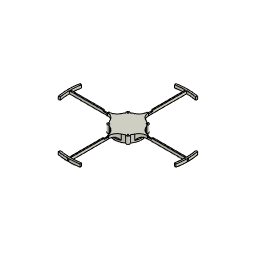
SoporteImán Nube Flotante v1 (Autodesk Fusion 360 design; units mm, degrees)
Autodesk Fusion 360 part; units mm, degrees
note: some values were not read from the file. Set by a fixed rule: which face or edge a step refers to.
sketch "Boceto1" plane through (0, 0, 0) normal (0, 0, 1) x (1, 0, 0)
  circle A0 centre (0, 0) radius 22.075
  circle A1 centre (0, 0) radius 24.075
  dimension "d1" = 44.15
  dimension "d2" = 2
  constraint coincident A0.centre A1.centre
  measures "d1" diameter of A0
extrude "Extruir1" add sketch "Boceto1" along normal blind 8 makes body 1
sketch "Boceto2" plane through (0, 0, 8) normal (0, 0, 1) x (-1, 0, 0)
  circle A0 centre (0, 0) radius 22.075
  circle A1 centre (0, 0) radius 24.075
  line L0 (0, 0) -> (-22.075, 0)
  line L1 (-22.075, 0) -> (-72.075, 0)
  line L2 (0, 0) -> (22.075, 0)
  line L3 (22.075, 0) -> (72.075, 0)
  line L4 (0, -22.075) -> (0, -72.075)
  line L5 (0, 22.075) -> (0, 72.075)
  line L6 (1, 22.075) -> (1, 72.075)
  line L7 (-1, 22.075) -> (-1, 72.075)
  line L8 (22.075, -1) -> (72.075, -1)
  line L9 (22.075, 1) -> (72.075, 1)
  line L10 (0, 1) -> (22.075, 1)
  line L11 (0, 1) -> (-22.075, 1)
  line L12 (-22.075, 1) -> (-72.075, 1)
  line L13 (-22.075, -1) -> (-72.075, -1)
  line L14 (1, -22.075) -> (1, -72.075)
  line L15 (-1, -22.075) -> (-1, -72.075)
  line L16 (72.075, 1) -> (72.075, -1)
  line L17 (1, 72.075) -> (-1, 72.075)
  line L18 (-72.075, 1) -> (-72.075, -1)
  line L19 (1, -72.075) -> (-1, -72.075)
  dimension "d7" = 50
  dimension "d8" = 50
  dimension "d9" = 50
  dimension "d10" = 50
  dimension "d11" = 1
  dimension "d12" = -1
  dimension "d13" = 1
  dimension "d14" = -1
  dimension "d15" = -1
  dimension "d16" = -1
  dimension "d17" = 1
  constraint coincident A0.centre A1.centre
  constraint coincident A0 L0.end
  constraint horizontal L0
  constraint parallel L0 L1
  constraint coincident A0 L2.end
  constraint parallel L0 L2
  constraint parallel L2 L3
  constraint coincident A0 L4.start
  constraint perpendicular L0 L4
  constraint coincident A0 L5.start
  constraint perpendicular L0 L5
  constraint perpendicular L8 L16
  constraint perpendicular L5 L17
  constraint perpendicular L13 L18
  constraint perpendicular L15 L19
  measures "d7" distance of L0.end L1.end
  measures "d8" distance of L2.end L3.end
  measures "d9" distance of L4.start L4.end
  measures "d10" distance of L5.start L5.end
extrude "Extruir2" add sketch "Boceto2" along normal blind 1 contours A0 L0 L2 | A0 A1 L1 L11 L12 | A0 L0 L2 L10 L11 | A0 A1 L1 L4 | A0 A1 L3 L4 | A0 A1 L5 L11 L12 | A0 L10 L11 | A0 A1 L3 L9 L10 | A0 A1 L5 L9 L10 bodies 1
extrude "Extruir4" add sketch "Boceto2" along normal blind 1 contours A1 L5 L6 L17 | A1 L5 L7 L17 bodies 1
extrude "Extruir5" add sketch "Boceto2" along normal blind 1 contours A1 L1 L12 L18 | A1 L1 L13 L18 | A1 L4 L15 L19 | A1 L4 L14 L19 | A1 L3 L8 L16 | A1 L3 L9 L16 bodies 1
sketch "Boceto3" plane through (0, 0, 9) normal (0, 0, 1) x (-1, 0, 0)
  arc A0 (-1, 24.0542) -> (-24.0542, 1) centre (0, 0) ccw
  line L0 (-24.0542, 1) -> (-72.075, 1)
  line L1 (-72.075, 1) -> (-72.075, -1)
  line L2 (-72.075, -1) -> (-24.0542, -1)
  arc A1 (-24.0542, -1) -> (-1, -24.0542) centre (0, 0) ccw
  line L3 (-1, -24.0542) -> (-1, -72.075)
  line L4 (-1, -72.075) -> (1, -72.075)
  line L5 (1, -72.075) -> (1, -24.0542)
  arc A2 (1, -24.0542) -> (24.0542, -1) centre (0, 0) ccw
  line L6 (24.0542, -1) -> (72.075, -1)
  line L7 (72.075, -1) -> (72.075, 1)
  line L8 (72.075, 1) -> (24.0542, 1)
  arc A3 (24.0542, 1) -> (1, 24.0542) centre (0, 0) ccw
  line L9 (1, 24.0542) -> (1, 72.075)
  line L10 (1, 72.075) -> (-1, 72.075)
  line L11 (-1, 72.075) -> (-1, 24.0542)
  circle A4 centre (0, 0) radius 24
  line L12 (0, 0) -> (16.2635, 16.2635)
  line L13 (0, 0) -> (23, 0) construction
  line L14 (16.2635, 16.2635) -> (-16.9706, -16.9706)
  line L15 (0, 0) -> (-16.9706, 16.9706)
  line L16 (-16.9706, 16.9706) -> (16.9706, -16.9706)
  circle A5 centre (-16.9706, 16.9706) radius 2
  circle A6 centre (16.2635, 16.2635) radius 2
  circle A7 centre (-16.9706, -16.9706) radius 2
  circle A8 centre (16.9706, -16.9706) radius 2
  dimension "d24" = 48
  dimension "d25" = 45
  dimension "d26" = 4
  dimension "d27" = 4
  dimension "d28" = 4
  dimension "d29" = 4
  constraint coincident A0.centre A1.centre
  constraint horizontal L13
  constraint coincident A4 L14.end
  constraint parallel L12 L14
  constraint coincident A4 L15.end
  constraint perpendicular L14 L15
  constraint coincident A4 L16.end
  constraint parallel L15 L16
  constraint coincident L15.end L16.start
  constraint coincident L12.end L14.start
  constraint coincident L14.end A7.centre
  constraint coincident L16.end A8.centre
  measures "d24" diameter of A4
  measures "d25" angle of L12 L13
  measures "d26" diameter of A5
  measures "d27" diameter of A6
  measures "d28" diameter of A7
  measures "d29" diameter of A8
extrude "Extruir6" add sketch "Boceto3" against normal blind 9 contours A0 A5 | A3 A6 | A1 A7 | A2 A8 bodies 1
sketch "Boceto4" plane through (0, 0, 9) normal (0, 0, 1) x (-1, 0, 0)
  arc A0 (-1, 24.0542) -> (-15.5506, 18.379) centre (0, 0) ccw
  arc A1 (-15.5506, 18.379) -> (-18.379, 15.5506) centre (-16.9706, 16.9706) ccw
  arc A2 (-18.379, 15.5506) -> (-24.0542, 1) centre (0, 0) ccw
  line L0 (-24.0542, 1) -> (-72.075, 1)
  line L1 (-72.075, 1) -> (-72.075, -1)
  line L2 (-72.075, -1) -> (-24.0542, -1)
  arc A3 (-24.0542, -1) -> (-18.379, -15.5506) centre (0, 0) ccw
  arc A4 (-18.379, -15.5506) -> (-15.5506, -18.379) centre (-16.9706, -16.9706) ccw
  arc A5 (-15.5506, -18.379) -> (-1, -24.0542) centre (0, 0) ccw
  line L3 (-1, -24.0542) -> (-1, -72.075)
  line L4 (-1, -72.075) -> (1, -72.075)
  line L5 (1, -72.075) -> (1, -24.0542)
  arc A6 (1, -24.0542) -> (15.5506, -18.379) centre (0, 0) ccw
  arc A7 (15.5506, -18.379) -> (18.379, -15.5506) centre (16.9706, -16.9706) ccw
  arc A8 (18.379, -15.5506) -> (24.0542, -1) centre (0, 0) ccw
  line L6 (24.0542, -1) -> (72.075, -1)
  line L7 (72.075, -1) -> (72.075, 1)
  line L8 (72.075, 1) -> (24.0542, 1)
  arc A9 (24.0542, 1) -> (18.1992, 15.7605) centre (0, 0) ccw
  arc A10 (18.1992, 15.7605) -> (15.7605, 18.1992) centre (16.2635, 16.2635) ccw
  arc A11 (15.7605, 18.1992) -> (1, 24.0542) centre (0, 0) ccw
  line L9 (1, 24.0542) -> (1, 72.075)
  line L10 (1, 72.075) -> (-1, 72.075)
  line L11 (-1, 72.075) -> (-1, 24.0542)
  circle A12 centre (-16.9706, -16.9706) radius 1.05
  circle A13 centre (16.9706, -16.9706) radius 1.05
  circle A14 centre (16.2635, 16.2635) radius 1.05
  circle A15 centre (-16.9706, 16.9706) radius 1.05
  dimension "d32" = 2.1
  dimension "d33" = 2.1
  dimension "d34" = 2.1
  dimension "d35" = 2.1
  constraint concentric A4 A12
  constraint concentric A7 A13
  constraint concentric A10 A14
  constraint concentric A1 A15
  measures "d32" diameter of A12
  measures "d33" diameter of A13
  measures "d34" diameter of A14
  measures "d35" diameter of A15
extrude "Extruir7" cut sketch "Boceto4" against normal blind 8 contours A12 | A13 | A14 | A15 bodies 1
extrude "Extruir8" add 1 faces at (-16.0835, -16.0654, 1) along direction (0, 0, 1) blind 120 separate body on bodies 1 makes body 2
extrude "Extruir9" add 1 faces at (-17.2533, 17.0815, 1) along direction (0, 0, 1) blind 120 separate body on bodies 1 makes body 3
extrude "Extruir10" add 1 faces at (16.6878, 17.0815, 1) along direction (0, 0, 1) blind 120 separate body on bodies 1 makes body 4
extrude "Extruir11" add 1 faces at (16.6878, -16.8596, 1) along direction (0, 0, 1) blind 120 separate body on bodies 1 makes body 5
sketch "Boceto5" plane through (0, 0, 9) normal (0, 0, 1) x (-1, 0, 0)
  circle A0 centre (-16.9706, -16.9706) radius 1.05
  circle A1 centre (16.9706, -16.9706) radius 1.05
  circle A2 centre (-16.9706, 16.9706) radius 1.05
  circle A3 centre (16.2635, 16.2635) radius 1.05
  arc A4 (-1, 24.0542) -> (-15.5506, 18.379) centre (0, 0) ccw
  arc A5 (-15.5506, 18.379) -> (-18.379, 15.5506) centre (-16.9706, 16.9706) ccw
  arc A6 (-18.379, 15.5506) -> (-24.0542, 1) centre (0, 0) ccw
  line L0 (-24.0542, 1) -> (-72.075, 1)
  line L1 (-72.075, 1) -> (-72.075, -1)
  line L2 (-72.075, -1) -> (-24.0542, -1)
  arc A7 (-24.0542, -1) -> (-18.379, -15.5506) centre (0, 0) ccw
  arc A8 (-18.379, -15.5506) -> (-15.5506, -18.379) centre (-16.9706, -16.9706) ccw
  arc A9 (-15.5506, -18.379) -> (-1, -24.0542) centre (0, 0) ccw
  line L3 (-1, -24.0542) -> (-1, -72.075)
  line L4 (-1, -72.075) -> (1, -72.075)
  line L5 (1, -72.075) -> (1, -24.0542)
  arc A10 (1, -24.0542) -> (15.5506, -18.379) centre (0, 0) ccw
  arc A11 (15.5506, -18.379) -> (18.379, -15.5506) centre (16.9706, -16.9706) ccw
  arc A12 (18.379, -15.5506) -> (24.0542, -1) centre (0, 0) ccw
  line L6 (24.0542, -1) -> (72.075, -1)
  line L7 (72.075, -1) -> (72.075, 1)
  line L8 (72.075, 1) -> (24.0542, 1)
  arc A13 (24.0542, 1) -> (18.1992, 15.7605) centre (0, 0) ccw
  arc A14 (18.1992, 15.7605) -> (15.7605, 18.1992) centre (16.2635, 16.2635) ccw
  arc A15 (15.7605, 18.1992) -> (1, 24.0542) centre (0, 0) ccw
  line L9 (1, 24.0542) -> (1, 72.075)
  line L10 (1, 72.075) -> (-1, 72.075)
  line L11 (-1, 72.075) -> (-1, 24.0542)
  circle A16 centre (0, 0) radius 24.075
  constraint coincident A4.centre A6.centre
  constraint coincident A11.end A16
extrude "Extruir12" add sketch "Boceto5" along normal blind 1 separate body contours A0 A1 A2 A4 A6 A7 A9 A10 A12 A13 A15 A16 | A0 A8 A16 | A2 A5 A16 | A1 A11 A16 | A14 A16 makes body 6
move_body "Desplazar1" bodies 6 to x (1, 0, 0) y (0, 1, 0) z (0, 0, 1) at (0, 0, 100)
sketch "Boceto6" plane through (0, 0, 110) normal (0, 0, 1) x (-1, 0, 0)
  circle A0 centre (-16.9706, 16.9706) radius 1.05
  circle A1 centre (16.2635, 16.2635) radius 1.05
  circle A2 centre (-16.9706, -16.9706) radius 1.05
  circle A3 centre (16.9706, -16.9706) radius 1.05
  arc A4 (18.379, -15.5506) -> (18.1992, 15.7605) centre (0, 0) ccw
  arc A5 (18.1992, 15.7605) -> (15.7605, 18.1992) centre (16.2635, 16.2635) ccw
  arc A6 (15.7605, 18.1992) -> (-15.5506, 18.379) centre (0, 0) ccw
  arc A7 (-15.5506, 18.379) -> (-18.379, 15.5506) centre (-16.9706, 16.9706) ccw
  arc A8 (-18.379, 15.5506) -> (-18.379, -15.5506) centre (0, 0) ccw
  arc A9 (-18.379, -15.5506) -> (-15.5506, -18.379) centre (-16.9706, -16.9706) ccw
  arc A10 (-15.5506, -18.379) -> (15.5506, -18.379) centre (0, 0) ccw
  arc A11 (15.5506, -18.379) -> (18.379, -15.5506) centre (16.9706, -16.9706) ccw
  circle A12 centre (0, 0) radius 20
  dimension "d48" = 40
  constraint coincident A4.centre A6.centre
  measures "d48" diameter of A12
extrude "Extruir13" cut sketch "Boceto6" against normal blind 1 contours A12 bodies 6
fillet "Empalme1" radius 15 1 edges at (-24.0542, 1, 8.5) on bodies 1
fillet "Empalme2" radius 15 1 edges at (-24.0542, -1, 8.5) on bodies 1
fillet "Empalme3" radius 15 2 edges at (-1, 24.0542, 8.5) (1, 24.0542, 8.5) on bodies 1
fillet "Empalme4" radius 15 4 edges at (24.0542, 1, 8.5) (24.0542, -1, 8.5) (1, -24.0542, 8.5) (-1, -24.0542, 8.5) on bodies 1
extrude "Extruir14" add 1 faces at (72.075, -0.3333, 8.3333) along direction (1, 0, 0) blind 20 on bodies 1 bodies 1
extrude "Extruir15" add 1 faces at (-0.3333, -72.075, 8.3333) along direction (0, -1, 0) blind 20 on bodies 1 bodies 1
extrude "Extruir16" add 1 faces at (-72.075, -0.3333, 8.3333) along direction (-1, 0, 0) blind 20 on bodies 1 bodies 1
extrude "Extruir17" add 1 faces at (-0.3333, 72.075, 8.3333) along direction (0, 1, 0) blind 20 on bodies 1 bodies 1
fillet "Empalme5" radius 5 1 edges at (-24.075, 0, 8) on bodies 1
fillet "Empalme6" radius 5 1 edges at (0, -24.075, 8) on bodies 1
fillet "Empalme7" radius 5 1 edges at (24.075, 0, 8) on bodies 1
fillet "Empalme8" radius 5 1 edges at (0, 24.075, 8) on bodies 1
extrude "Extruir18" add 1 faces at (-5.096, 5.6045, 9) along direction (0, 0, 1) blind 2 on bodies 1 bodies 1
sketch "Boceto7" plane through (0, 0, 11) normal (0, 0, 1) x (-1, 0, 0)
  circle A0 centre (-16.9706, -16.9706) radius 1.05
  circle A1 centre (16.9706, -16.9706) radius 1.05
  circle A2 centre (-16.9706, 16.9706) radius 1.05
  circle A3 centre (16.2635, 16.2635) radius 1.05
  arc A4 (-9.858, 21.9642) -> (-15.5506, 18.379) centre (0, 0) ccw
  arc A5 (-15.5506, 18.379) -> (-18.379, 15.5506) centre (-16.9706, 16.9706) ccw
  arc A6 (-18.379, 15.5506) -> (-21.9642, 9.858) centre (0, 0) ccw
  arc A7 (-35.6491, 1) -> (-21.9642, 9.858) centre (-35.6491, 16) ccw
  line L0 (-35.6491, 1) -> (-92.075, 1)
  line L1 (-92.075, 1) -> (-92.075, -1)
  line L2 (-92.075, -1) -> (-35.6491, -1)
  arc A8 (-21.9642, -9.858) -> (-35.6491, -1) centre (-35.6491, -16) ccw
  arc A9 (-21.9642, -9.858) -> (-18.379, -15.5506) centre (0, 0) ccw
  arc A10 (-18.379, -15.5506) -> (-15.5506, -18.379) centre (-16.9706, -16.9706) ccw
  arc A11 (-15.5506, -18.379) -> (-9.858, -21.9642) centre (0, 0) ccw
  arc A12 (-1, -35.6491) -> (-9.858, -21.9642) centre (-16, -35.6491) ccw
  line L3 (-1, -35.6491) -> (-1, -92.075)
  line L4 (-1, -92.075) -> (1, -92.075)
  line L5 (1, -92.075) -> (1, -35.6491)
  arc A13 (9.858, -21.9642) -> (1, -35.6491) centre (16, -35.6491) ccw
  arc A14 (9.858, -21.9642) -> (15.5506, -18.379) centre (0, 0) ccw
  arc A15 (15.5506, -18.379) -> (18.379, -15.5506) centre (16.9706, -16.9706) ccw
  arc A16 (18.379, -15.5506) -> (21.9642, -9.858) centre (0, 0) ccw
  arc A17 (35.6491, -1) -> (21.9642, -9.858) centre (35.6491, -16) ccw
  line L6 (35.6491, -1) -> (92.075, -1)
  line L7 (92.075, -1) -> (92.075, 1)
  line L8 (92.075, 1) -> (35.6491, 1)
  arc A18 (21.9642, 9.858) -> (35.6491, 1) centre (35.6491, 16) ccw
  arc A19 (21.9642, 9.858) -> (18.1992, 15.7605) centre (0, 0) ccw
  arc A20 (18.1992, 15.7605) -> (15.7605, 18.1992) centre (16.2635, 16.2635) ccw
  arc A21 (15.7605, 18.1992) -> (9.858, 21.9642) centre (0, 0) ccw
  arc A22 (1, 35.6491) -> (9.858, 21.9642) centre (16, 35.6491) ccw
  line L9 (1, 35.6491) -> (1, 92.075)
  line L10 (1, 92.075) -> (-1, 92.075)
  line L11 (-1, 92.075) -> (-1, 35.6491)
  arc A23 (-9.858, 21.9642) -> (-1, 35.6491) centre (-16, 35.6491) ccw
  circle A24 centre (16.9706, -16.9706) radius 3
  circle A25 centre (16.2635, 16.2635) radius 3
  circle A26 centre (-16.9706, -16.9706) radius 3
  circle A27 centre (-16.9706, 16.9706) radius 3
  circle A28 centre (16.9706, -16.9706) radius 1.15
  circle A29 centre (16.2635, 16.2635) radius 1.15
  circle A30 centre (-16.9706, 16.9706) radius 1.15
  circle A31 centre (-16.9706, -16.9706) radius 1.15
  dimension "d77" = 6
  dimension "d78" = 6
  dimension "d79" = 6
  dimension "d80" = 6
  dimension "d83" = 0.1
  dimension "d84" = 0.1
  dimension "d85" = 0.1
  dimension "d86" = 0.1
  constraint concentric A1 A24
  constraint concentric A3 A25
  constraint concentric A0 A26
  constraint concentric A2 A27
  measures "d77" diameter of A24
  measures "d78" diameter of A25
  measures "d79" diameter of A26
  measures "d80" diameter of A27
extrude "Extruir19" add sketch "Boceto7" against normal blind 11 contours A4 A5 A6 A27 | A19 A20 A21 A25 | A9 A10 A11 A26 | A14 A15 A16 A24 picked at (-18.9089, 15.5078) picked at (18.6467, 15.8095) picked at (-15.5078, -18.9089) picked at (18.8996, -15.4923) bodies 1
sketch "Boceto8" plane through (0, 0, 0) normal (0, 0, -1) x (1, 0, 0)
  circle A0 centre (0, 0) radius 22.075
  arc A1 (14.7713, -19.0109) -> (19.0109, -14.7713) centre (16.9706, -16.9706) ccw
  arc A2 (19.0109, -14.7713) -> (19.0109, 14.7713) centre (0, 0) ccw
  arc A3 (19.0109, 14.7713) -> (14.7713, 19.0109) centre (16.9706, 16.9706) ccw
  arc A4 (14.7713, 19.0109) -> (-14.8804, 18.9256) centre (0, 0) ccw
  arc A5 (-14.8804, 18.9256) -> (-18.9256, 14.8804) centre (-16.2635, 16.2635) ccw
  arc A6 (-18.9256, 14.8804) -> (-19.0109, -14.7713) centre (0, 0) ccw
  arc A7 (-19.0109, -14.7713) -> (-14.7713, -19.0109) centre (-16.9706, -16.9706) ccw
  arc A8 (-14.7713, -19.0109) -> (14.7713, -19.0109) centre (0, 0) ccw
  circle A9 centre (0, 0) radius 24.0416
extrude "Extruir21" add 5 faces at (16.7039, 16.3148, 0) (15.5078, 18.9089, 0) (-15.5078, 18.9089, 0) (-15.7484, -18.6375, 0) (15.5078, -18.9089, 0) along direction (0, 0, 1) blind 11 on bodies 1 bodies 1
sketch "Boceto9" plane through (0, 0, 0) normal (0, 0, -1) x (1, 0, 0)
  circle A0 centre (0, 0) radius 22.075
  arc A1 (14.7713, -19.0109) -> (19.0109, -14.7713) centre (16.9706, -16.9706) ccw
  arc A2 (19.0109, -14.7713) -> (19.0109, 14.7713) centre (0, 0) ccw
  arc A3 (19.0109, 14.7713) -> (14.7713, 19.0109) centre (16.9706, 16.9706) ccw
  arc A4 (14.7713, 19.0109) -> (-14.8804, 18.9256) centre (0, 0) ccw
  arc A5 (-14.8804, 18.9256) -> (-18.9256, 14.8804) centre (-16.2635, 16.2635) ccw
  arc A6 (-18.9256, 14.8804) -> (-19.0109, -14.7713) centre (0, 0) ccw
  arc A7 (-19.0109, -14.7713) -> (-14.7713, -19.0109) centre (-16.9706, -16.9706) ccw
  arc A8 (-14.7713, -19.0109) -> (14.7713, -19.0109) centre (0, 0) ccw
  circle A9 centre (0, 0) radius 24
  line L0 (0, 0) -> (-16.9706, 16.9706)
  line L1 (0, 0) -> (24, 0) construction
  circle A10 centre (-16.9706, 16.9706) radius 3
  dimension "d91" = 135
  dimension "d92" = 6
  constraint concentric A0 A9
  constraint coincident A3.centre A9
  constraint horizontal L1
  constraint coincident A0.centre A2.centre
  constraint coincident L0.end A10.centre
  measures "d91" angle of L0 L1
  measures "d92" diameter of A10
extrude "Extruir22" add sketch "Boceto9" against normal blind 11 contours A4 A5 A6 A10 bodies 1
sketch "Boceto10" plane through (0, 0, 11) normal (0, 0, 1) x (-1, 0, 0)
  arc A0 (1, 35.6491) -> (9.858, 21.9642) centre (16, 35.6491) ccw
  line L0 (1, 35.6491) -> (1, 92.075)
  line L1 (1, 92.075) -> (-1, 92.075)
  line L2 (-1, 92.075) -> (-1, 35.6491)
  arc A1 (-9.858, 21.9642) -> (-1, 35.6491) centre (-16, 35.6491) ccw
  arc A2 (-9.858, 21.9642) -> (-14.7713, 19.0109) centre (0, 0) ccw
  arc A3 (-14.7713, 19.0109) -> (-19.0109, 14.7713) centre (-16.9706, 16.9706) ccw
  arc A4 (-19.0109, 14.7713) -> (-21.9642, 9.858) centre (0, 0) ccw
  arc A5 (-35.6491, 1) -> (-21.9642, 9.858) centre (-35.6491, 16) ccw
  line L3 (-35.6491, 1) -> (-92.075, 1)
  line L4 (-92.075, 1) -> (-92.075, -1)
  line L5 (-92.075, -1) -> (-35.6491, -1)
  arc A6 (-21.9642, -9.858) -> (-35.6491, -1) centre (-35.6491, -16) ccw
  arc A7 (-21.9642, -9.858) -> (-19.0109, -14.7713) centre (0, 0) ccw
  arc A8 (-19.0109, -14.7713) -> (-14.7713, -19.0109) centre (-16.9706, -16.9706) ccw
  arc A9 (-14.7713, -19.0109) -> (-9.858, -21.9642) centre (0, 0) ccw
  arc A10 (-1, -35.6491) -> (-9.858, -21.9642) centre (-16, -35.6491) ccw
  line L6 (-1, -35.6491) -> (-1, -92.075)
  line L7 (-1, -92.075) -> (1, -92.075)
  line L8 (1, -92.075) -> (1, -35.6491)
  arc A11 (9.858, -21.9642) -> (1, -35.6491) centre (16, -35.6491) ccw
  arc A12 (9.858, -21.9642) -> (14.7713, -19.0109) centre (0, 0) ccw
  arc A13 (14.7713, -19.0109) -> (19.0109, -14.7713) centre (16.9706, -16.9706) ccw
  arc A14 (19.0109, -14.7713) -> (21.9642, -9.858) centre (0, 0) ccw
  arc A15 (35.6491, -1) -> (21.9642, -9.858) centre (35.6491, -16) ccw
  line L9 (35.6491, -1) -> (92.075, -1)
  line L10 (92.075, -1) -> (92.075, 1)
  line L11 (92.075, 1) -> (35.6491, 1)
  arc A16 (21.9642, 9.858) -> (35.6491, 1) centre (35.6491, 16) ccw
  arc A17 (21.9642, 9.858) -> (19.0109, 14.7713) centre (0, 0) ccw
  arc A18 (19.0109, 14.7713) -> (14.7713, 19.0109) centre (16.9706, 16.9706) ccw
  arc A19 (14.7713, 19.0109) -> (9.858, 21.9642) centre (0, 0) ccw
  arc A20 (15.9498, 15.2614) -> (15.2614, 15.9498) centre (0, 0) ccw
  arc A21 (15.2614, 15.9498) -> (15.9498, 15.2614) centre (16.2635, 16.2635) ccw
extrude "Extruir23" add sketch "Boceto10" against normal blind 3 contours A20 A21 bodies 1
sketch "Boceto11" plane through (0, 0, 11) normal (0, 0, 1) x (-1, 0, 0)
  arc A0 (1, 35.6491) -> (9.858, 21.9642) centre (16, 35.6491) ccw
  line L0 (1, 35.6491) -> (1, 92.075)
  line L1 (1, 92.075) -> (-1, 92.075)
  line L2 (-1, 92.075) -> (-1, 35.6491)
  arc A1 (-9.858, 21.9642) -> (-1, 35.6491) centre (-16, 35.6491) ccw
  arc A2 (-9.858, 21.9642) -> (-14.7713, 19.0109) centre (0, 0) ccw
  arc A3 (-14.7713, 19.0109) -> (-19.0109, 14.7713) centre (-16.9706, 16.9706) ccw
  arc A4 (-19.0109, 14.7713) -> (-21.9642, 9.858) centre (0, 0) ccw
  arc A5 (-35.6491, 1) -> (-21.9642, 9.858) centre (-35.6491, 16) ccw
  line L3 (-35.6491, 1) -> (-92.075, 1)
  line L4 (-92.075, 1) -> (-92.075, -1)
  line L5 (-92.075, -1) -> (-35.6491, -1)
  arc A6 (-21.9642, -9.858) -> (-35.6491, -1) centre (-35.6491, -16) ccw
  arc A7 (-21.9642, -9.858) -> (-19.0109, -14.7713) centre (0, 0) ccw
  arc A8 (-19.0109, -14.7713) -> (-14.7713, -19.0109) centre (-16.9706, -16.9706) ccw
  arc A9 (-14.7713, -19.0109) -> (-9.858, -21.9642) centre (0, 0) ccw
  arc A10 (-1, -35.6491) -> (-9.858, -21.9642) centre (-16, -35.6491) ccw
  line L6 (-1, -35.6491) -> (-1, -92.075)
  line L7 (-1, -92.075) -> (1, -92.075)
  line L8 (1, -92.075) -> (1, -35.6491)
  arc A11 (9.858, -21.9642) -> (1, -35.6491) centre (16, -35.6491) ccw
  arc A12 (9.858, -21.9642) -> (14.7713, -19.0109) centre (0, 0) ccw
  arc A13 (14.7713, -19.0109) -> (19.0109, -14.7713) centre (16.9706, -16.9706) ccw
  arc A14 (19.0109, -14.7713) -> (21.9642, -9.858) centre (0, 0) ccw
  arc A15 (35.6491, -1) -> (21.9642, -9.858) centre (35.6491, -16) ccw
  line L9 (35.6491, -1) -> (92.075, -1)
  line L10 (92.075, -1) -> (92.075, 1)
  line L11 (92.075, 1) -> (35.6491, 1)
  arc A16 (21.9642, 9.858) -> (35.6491, 1) centre (35.6491, 16) ccw
  arc A17 (21.9642, 9.858) -> (19.0109, 14.7713) centre (0, 0) ccw
  arc A18 (19.0109, 14.7713) -> (14.7713, 19.0109) centre (16.9706, 16.9706) ccw
  arc A19 (14.7713, 19.0109) -> (9.858, 21.9642) centre (0, 0) ccw
  circle A20 centre (0, 0) radius 24 construction
  circle A21 centre (-16.9706, -16.9706) radius 1.075
  circle A22 centre (16.9706, -16.9706) radius 1.075
  circle A23 centre (16.9706, 16.9706) radius 1.075
  circle A24 centre (-16.9706, 16.9706) radius 1.075
  dimension "d97" = 2.15
  dimension "d99" = 360
  constraint coincident A2.centre A4.centre
  constraint coincident A8.centre A20
  constraint concentric A8 A21
  measures "d97" diameter of A21
extrude "Extruir24" cut sketch "Boceto11" against normal blind 10 contours A21 | A22 | A23 | A24 bodies 1
extrude "Extruir25" add 13 faces at (-15.5973, -15.5632, 11) (5.0829, 5.3256, 11) (-15.5963, -16.0684, 11) (17.9637, -13.8819, 11) (-15.5078, 18.9089, 11) (-27.6146, 0, 11) (-18.6166, -18.6166, 11) (-15.7339, -18.6358, 11) (0, -27.6146, 11) (18.9089, -15.5078, 11) (27.6146, 0, 11) (18.9089, 15.5078, 11) (0, 27.6146, 11) along direction (0, 0, 1) blind 1 on bodies 1 bodies 1
sketch "Boceto12" plane through (0, 0, 12) normal (0, 0, 1) x (-1, 0, 0)
  circle A0 centre (16.9706, -16.9706) radius 1.075
  circle A1 centre (16.9706, 16.9706) radius 1.075
  circle A2 centre (-16.9706, -16.9706) radius 1.075
  circle A3 centre (-16.9706, 16.9706) radius 1.075
  arc A4 (1, 35.6491) -> (9.858, 21.9642) centre (16, 35.6491) ccw
  line L0 (1, 35.6491) -> (1, 92.075)
  line L1 (1, 92.075) -> (-1, 92.075)
  line L2 (-1, 92.075) -> (-1, 35.6491)
  arc A5 (-9.858, 21.9642) -> (-1, 35.6491) centre (-16, 35.6491) ccw
  arc A6 (-9.858, 21.9642) -> (-14.7713, 19.0109) centre (0, 0) ccw
  arc A7 (-14.7713, 19.0109) -> (-19.0109, 14.7713) centre (-16.9706, 16.9706) ccw
  arc A8 (-19.0109, 14.7713) -> (-21.9642, 9.858) centre (0, 0) ccw
  arc A9 (-35.6491, 1) -> (-21.9642, 9.858) centre (-35.6491, 16) ccw
  line L3 (-35.6491, 1) -> (-92.075, 1)
  line L4 (-92.075, 1) -> (-92.075, -1)
  line L5 (-92.075, -1) -> (-35.6491, -1)
  arc A10 (-21.9642, -9.858) -> (-35.6491, -1) centre (-35.6491, -16) ccw
  arc A11 (-21.9642, -9.858) -> (-19.0109, -14.7713) centre (0, 0) ccw
  arc A12 (-19.0109, -14.7713) -> (-14.7713, -19.0109) centre (-16.9706, -16.9706) ccw
  arc A13 (-14.7713, -19.0109) -> (-9.858, -21.9642) centre (0, 0) ccw
  arc A14 (-1, -35.6491) -> (-9.858, -21.9642) centre (-16, -35.6491) ccw
  line L6 (-1, -35.6491) -> (-1, -92.075)
  line L7 (-1, -92.075) -> (1, -92.075)
  line L8 (1, -92.075) -> (1, -35.6491)
  arc A15 (9.858, -21.9642) -> (1, -35.6491) centre (16, -35.6491) ccw
  arc A16 (9.858, -21.9642) -> (14.7713, -19.0109) centre (0, 0) ccw
  arc A17 (14.7713, -19.0109) -> (19.0109, -14.7713) centre (16.9706, -16.9706) ccw
  arc A18 (19.0109, -14.7713) -> (21.9642, -9.858) centre (0, 0) ccw
  arc A19 (35.6491, -1) -> (21.9642, -9.858) centre (35.6491, -16) ccw
  line L9 (35.6491, -1) -> (92.075, -1)
  line L10 (92.075, -1) -> (92.075, 1)
  line L11 (92.075, 1) -> (35.6491, 1)
  arc A20 (21.9642, 9.858) -> (35.6491, 1) centre (35.6491, 16) ccw
  arc A21 (21.9642, 9.858) -> (19.0109, 14.7713) centre (0, 0) ccw
  arc A22 (19.0109, 14.7713) -> (14.7713, 19.0109) centre (16.9706, 16.9706) ccw
  arc A23 (14.7713, 19.0109) -> (9.858, 21.9642) centre (0, 0) ccw
  circle A24 centre (0, 0) radius 43.5
  circle A25 centre (0, 0) radius 35.5
  dimension "d104" = 87
  dimension "d105" = 71
  constraint concentric A6 A24
  constraint coincident A6.centre A8.centre
  measures "d104" diameter of A24
  measures "d105" diameter of A25
extrude "Extruir26" cut sketch "Boceto12" against normal blind 1 contours A4 L0 L2 A5 A24 A25 | A19 L9 L11 A20 A24 A25 | A9 L3 L5 A10 A24 A25 | A14 L6 L8 A15 A24 A25 bodies 1
extrude "Extruir27" add 5 faces at (0.1111, -75.8829, 12) (75.8829, -0.1111, 12) (5.3806, -5.4035, 12) (-75.8829, -0.1111, 12) (0.1111, 75.8829, 12) along direction (0, 0, 1) blind 1 on bodies 1 bodies 1
extrude "Extruir28" add 4 faces at (92.075, 0.3333, 9.6667) (92.075, -0.3333, 8.3333) (92.075, 0.3333, 11.3333) (92.075, 0.3333, 12.3333) along direction (1, 0, 0) blind 15 on bodies 1 bodies 1
extrude "Extruir29" add 4 faces at (-0.3333, 92.075, 9.6667) (-0.3333, 92.075, 8.3333) (-0.3333, 92.075, 11.3333) (-0.3333, 92.075, 12.3333) along direction (0, 1, 0) blind 15 on bodies 1 bodies 1
extrude "Extruir30" add 4 faces at (-92.075, -0.3333, 9.6667) (-92.075, -0.3333, 8.3333) (-92.075, -0.3333, 11.3333) (-92.075, -0.3333, 12.3333) along direction (-1, 0, 0) blind 15 on bodies 1 bodies 1
extrude "Extruir31" add 4 faces at (-0.3333, -92.075, 8.3333) (0.3333, -92.075, 9.6667) (0.3333, -92.075, 11.3333) (0.3333, -92.075, 12.3333) along direction (0, -1, 0) blind 15 on bodies 1 bodies 1
sketch "Boceto13" plane through (0, 0, 0) normal (0, 0, -1) x (1, 0, 0)
  circle A0 centre (0, 0) radius 22.075
  arc A1 (14.7713, -19.0109) -> (19.0109, -14.7713) centre (16.9706, -16.9706) ccw
  arc A2 (19.0109, -14.7713) -> (19.0109, 14.7713) centre (0, 0) ccw
  arc A3 (19.0109, 14.7713) -> (14.7713, 19.0109) centre (16.9706, 16.9706) ccw
  arc A4 (14.7713, 19.0109) -> (-14.7713, 19.0109) centre (0, 0) ccw
  arc A5 (-14.7713, 19.0109) -> (-19.0109, 14.7713) centre (-16.9706, 16.9706) ccw
  arc A6 (-19.0109, 14.7713) -> (-19.0109, -14.7713) centre (0, 0) ccw
  arc A7 (-19.0109, -14.7713) -> (-14.7713, -19.0109) centre (-16.9706, -16.9706) ccw
  arc A8 (-14.7713, -19.0109) -> (14.7713, -19.0109) centre (0, 0) ccw
  circle A9 centre (0, 0) radius 21.975
  dimension "d118" = -0.1
extrude "Extruir32" add sketch "Boceto13" against normal blind 8 contours A0 bodies 1
sketch "Boceto14" plane through (0, 0, 13) normal (0, 0, 1) x (-1, 0, 0)
  arc A0 (-43.4885, 1) -> (-43.4885, -1) centre (0, 0) ccw
  line L0 (-43.4885, 1) -> (-107.075, 1)
  line L1 (-107.075, 1) -> (-107.075, -1)
  line L2 (-107.075, -1) -> (-43.4885, -1)
  arc A1 (-105.2746, 19.5782) -> (-107.075, 1) centre (0, 0) ccw
  line L3 (0, 0) -> (-105.2746, 19.5782) construction
  line L4 (0, 0) -> (-107.075, 1) construction
  arc A2 (-107.075, -1) -> (-105.2746, -19.5782) centre (0, 0) ccw
  line L5 (0, 0) -> (-107.075, -1) construction
  line L6 (0, 0) -> (-105.2746, -19.5782) construction
  line L7 (-105.2746, -19.5782) -> (-102.3252, -19.0297)
  line L8 (-107.075, -1) -> (-104.0751, -0.972)
  arc A3 (-104.0751, -0.972) -> (-102.3252, -19.0297) centre (0, 0) ccw
  arc A4 (-102.2516, 19.016) -> (-104, 1) centre (0, 0) ccw
  line L9 (-105.2746, 19.5782) -> (-102.2516, 19.016)
  line L10 (-19.5782, -105.2746) -> (-19.016, -102.2516)
  arc A5 (-19.5782, -105.2746) -> (-1, -107.075) centre (0, 0) ccw
  line L11 (0, 0) -> (-1, -107.075) construction
  arc A6 (-19.016, -102.2516) -> (-1, -104) centre (0, 0) ccw
  line L12 (0, 0) -> (1, -107.075) construction
  arc A7 (0.972, -104.0751) -> (19.0297, -102.3252) centre (0, 0) ccw
  arc A8 (1, -107.075) -> (19.5782, -105.2746) centre (0, 0) ccw
  line L13 (19.5782, -105.2746) -> (19.0297, -102.3252)
  line L14 (105.2746, -19.5782) -> (102.2516, -19.016)
  arc A9 (105.2746, -19.5782) -> (107.075, -1) centre (0, 0) ccw
  line L15 (0, 0) -> (107.075, -1) construction
  arc A10 (102.2516, -19.016) -> (104, -1) centre (0, 0) ccw
  line L16 (0, 0) -> (107.075, 1) construction
  arc A11 (104.0751, 0.972) -> (102.3252, 19.0297) centre (0, 0) ccw
  arc A12 (107.075, 1) -> (105.2746, 19.5782) centre (0, 0) ccw
  line L17 (105.2746, 19.5782) -> (102.3252, 19.0297)
  line L18 (19.5782, 105.2746) -> (19.016, 102.2516)
  arc A13 (19.5782, 105.2746) -> (1, 107.075) centre (0, 0) ccw
  line L19 (0, 0) -> (1, 107.075) construction
  arc A14 (19.016, 102.2516) -> (1, 104) centre (0, 0) ccw
  line L20 (0, 0) -> (-1, 107.075) construction
  arc A15 (-0.972, 104.0751) -> (-19.0297, 102.3252) centre (0, 0) ccw
  arc A16 (-1, 107.075) -> (-19.5782, 105.2746) centre (0, 0) ccw
  line L21 (-19.5782, 105.2746) -> (-19.0297, 102.3252)
  line L22 (1, -107.075) -> (0.972, -104.0751)
  line L23 (-1, -104) -> (-1, -107.075)
  line L24 (107.075, -1) -> (104, -1)
  line L25 (104.0751, 0.972) -> (107.075, 1)
  line L26 (-0.972, 104.0751) -> (-1, 107.075)
  line L27 (1, 104) -> (1, 107.075)
  dimension "d121" = 10
  dimension "d122" = 10
  dimension "d123" = 3
  dimension "d124" = 3
  dimension "d126" = 360
  constraint coincident L0.end L1.start
  constraint coincident A0.centre A1.centre
  constraint coincident L1.end L2.start
  constraint parallel L6 L7
  constraint parallel L5 L8
  constraint coincident L0 A4.end
  constraint parallel L3 L9
  constraint perpendicular L23 L24
  measures "d121" angle of L3 L4
  measures "d122" angle of L5 L6
  measures "d123" distance of A2.end L7.end
  measures "d124" distance of L1.end L8.end
extrude "Extruir33" add sketch "Boceto14" against normal blind 5 contours L0 A1 A4 L9 | L2 A2 L7 A3 | L10 A5 A6 L23 | A7 A8 L13 L22 | L14 A9 A10 L24 | A11 A12 L17 L25 | L18 A13 A14 L27 | A15 A16 L21 L26 bodies 1
extrude "Extruir20" [suppressed]
extrude "Extruir3" [suppressed]
hidden bodies 2 3 4 5 6
named bodies: "Soporte Imán", "Torre1", "Torre2", "Torre3", "Torre4", "Soporte torres"
